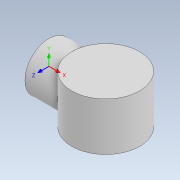
# Autodesk Inventor part: hip_inventor
Saved by Autodesk Inventor 2020 (Build 240168000, 168)
## iProperties
Created: 2021-01-07
Part Number: hip_inventor
Material: Generic
Document SubType Name: Modeling
Designer: DELL
Density: 1 g/cm^3
Appearance: Default
Author: DELL
Autodesk Inventor part; units mm, degrees
ref_plane "YZ Plane" through (0, 0, 0) normal (1, 0, 0) x (0, 1, 0)
ref_plane "XZ Plane" through (0, 0, 0) normal (0, 1, 0) x (-1, 0, 0)
ref_plane "XY Plane" through (0, 0, 0) normal (0, 0, 1) x (1, 0, 0)
sketch "Sketch1" plane through (0, 0, 0) normal (1, 0, 0) x (0, 1, 0)
  circle A0 centre (0, 0) radius 28
  dimension "d0" = 56
  constraints: 1 centre point, 1 coincident
  measures "d0" diameter of A0
extrude "Extrusion1" add sketch "Sketch1" along normal blind 66
sketch "Sketch2" plane through (0, 0, 0) normal (0, 1, 0) x (-1, 0, 0)
  line L0 (-66, 28) -> (-66, -28) projected
  circle A0 centre (-66, 0) radius 39.5
  point P0 (0, 0)
  dimension "d3" = 79
  constraints: 1 centre point, 1 midpoint
  measures "d3" diameter of A0
extrude "Extrusion2" add sketch "Sketch2" along normal mid plane 56
sketch "Sketch3" plane through (0, 0, 0) normal (0, 1, 0) x (-1, 0, 0)
  circle A0 centre (-66, 0) radius 39.5 projected
  circle A1 centre (-66, 0) radius 31.5
  circle A2 centre (-66, 0) radius 39.5
  point P0 (0, 0)
  point P1 (-26.5, 0)
  dimension "d12" = 79
  dimension "d13" = 63
  constraints: 2 centre point, 2 coincident, 1 horizontal alignment
  measures "d12" diameter of A2
  measures "d13" diameter of A1
body "Solid1"
